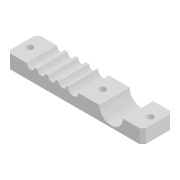
# Autodesk Inventor part: C_Unit_Cable_Holder_B
Saved by Autodesk Inventor 2020 (Build 240168000, 168)
## iProperties
Created: 2021-02-20
Part Number: C_Unit_Cable_Holder_B
Material: 一般
Document SubType Name: Modeling
Designer: ken113
Density: 1 g/cm^3
Appearance: 既定
Author: ken113
Autodesk Inventor part; units mm, degrees
ref_plane "YZ Plane" through (0, 0, 0) normal (1, 0, 0) x (0, 1, 0)
ref_plane "XZ Plane" through (0, 0, 0) normal (0, 1, 0) x (-1, 0, 0)
ref_plane "XY Plane" through (0, 0, 0) normal (0, 0, 1) x (1, 0, 0)
sketch "スケッチ1" plane through (0, 0, 0) normal (0, 0, 1) x (1, 0, 0)
  circle A0 centre (0, 9) radius 7.75
  line L0 (10.75, 0) -> (-58.5, 0)
  line L1 (-58.5, 0) -> (-58.5, 1.25)
  line L2 (-58.5, 1.25) -> (10.75, 1.25)
  line L3 (10.75, 1.25) -> (10.75, 0)
  circle A1 centre (0, 9) radius 10.75
  line L4 (10.75, 1.25) -> (10.75, 15.8822)
  circle A2 centre (-32, 9) radius 2.5
  circle A3 centre (-39, 9) radius 2.5
  circle A4 centre (-25, 9) radius 3.5
  circle A5 centre (-46, 9) radius 2.5
  circle A6 centre (-53, 9) radius 2.5
  circle A7 centre (-53, 9) radius 5.5
  line L5 (-58.5, 1.25) -> (-58.5, 21.0928)
  line L6 (-61.1769, 14.5) -> (16.6826, 14.5)
  point P0 (0, 0)
  point P1 (-9.2365, 14.5)
  point P2 (-58.5, 14.5)
  point P3 (10.75, 14.5)
  point P4 (9.2365, 14.5)
  point P5 (10.75, 9)
  point P6 (5.879, 0)
  point P7 (-5.879, 0)
  dimension "d0" = 15.5
  dimension "d1" = 3
  dimension "d2" = 5
  dimension "d3" = 5
  dimension "d4" = 7
  dimension "d5" = 5
  dimension "d7" = 7
  dimension "d8" = 7
  dimension "d9" = 25
  dimension "d10" = 7
  dimension "d11" = 5
  dimension "d12" = 7
  dimension "d13" = 3
  dimension "d16" = 9
  constraints: 14 end point, 8 centre point, 7 horizontal alignment, 6 tangent, 2 parallel, 2 perpendicular, 1 horizontal, 1 vertical alignment
  measures "d0" diameter of A0
  measures "d1" radial gap between concentric circles of A0 A1
  measures "d2" diameter of A2
  measures "d3" diameter of A3
  measures "d4" diameter of A4
  measures "d5" diameter of A5
  measures "d7" distance of A2.centre A3.centre
  measures "d8" distance of A5.centre A3.centre
  measures "d9" distance of A0.centre A4.centre
  measures "d10" distance of A4.centre A2.centre
  measures "d11" diameter of A6
  measures "d12" distance of A6.centre A5.centre
  measures "d13" radial gap between concentric circles of A6 A7
  measures "d16" distance from line of A4.centre L0
extrude "押し出し1" add sketch "スケッチ1" along normal blind 20 contours A0 L6 A1 L2 | A0 L6 A1 | L2 A1 L6 A0 | L2 A1 L0 | L6 L4 A1 | A1 L0 L1 L2 | L2 L5 A7 A5 L6 A1 | A1 L4 L2 | L2 L3 L0 A1 | A7 A5 | A7 L5 L6 picked at (-49.0972, 10.8197)
sketch "スケッチ3" plane through (0, 0, 20) normal (0, 0, 1) x (1, 0, 0)
  line L0 (-9.2365, 14.5) -> (-58.5, 14.5) projected
  line L1 (-58.5, 14.5) -> (-58.5, 0) projected
  line L2 (-58.5, 0) -> (10.75, 0) projected
  arc A0 (9.2365, 14.5) -> (-9.2365, 14.5) centre (0, 9) ccw projected
  circle A1 centre (0, 9) radius 7.75 projected
  circle A2 centre (-53, 9) radius 2.5 projected
  circle A3 centre (-25, 9) radius 3.5 projected
  circle A4 centre (-39, 9) radius 2.5 projected
  circle A5 centre (-32, 9) radius 2.5 projected
  circle A6 centre (-46, 9) radius 2.5 projected
  line L3 (-58.5, 14.5) -> (-58.5, 0) projected
  line L4 (-58.5, 0) -> (-68.5, 0)
  line L5 (-68.5, 0) -> (-68.5, 14.5)
  line L6 (-68.5, 14.5) -> (-58.5, 14.5)
  line L7 (-58.5, 14.5) -> (-58.5, 0)
  line L8 (10.75, -0.0065) -> (20.75, -0.0065)
  line L9 (20.75, -0.0065) -> (20.75, 14.5)
  line L10 (20.75, 14.5) -> (10.75, 14.5)
  line L11 (10.75, 14.5) -> (10.75, -0.0065)
  line L12 (10.75, 0) -> (10.75, 14.5) projected
  line L13 (10.75, 14.5) -> (9.2365, 14.5) projected
  point P0 (0, 0)
  dimension "d17" = 10
  dimension "d18" = 10
  constraints: 16 end point, 4 parallel, 2 horizontal, 2 perpendicular, 1 coincident, 1 horizontal alignment
  measures "d17" distance of L5.end L6.end
  measures "d18" distance of L10.end L9.end
extrude "押し出し2" add sketch "スケッチ3" against normal up to surface (20 mm away) contours L1 L4 L5 L6 | L10 L9 L8 L11
sketch "スケッチ4" plane through (0, 0, 20) normal (0, 0, 1) x (1, 0, 0)
  line L0 (-9.2365, 14.5) -> (-68.5, 14.5) projected
  line L1 (-68.5, 14.5) -> (-68.5, 0) projected
  line L2 (-68.5, 0) -> (10.75, 0) projected
  line L3 (20.75, -0.0065) -> (20.75, 14.5) projected
  line L4 (20.75, 14.5) -> (9.2365, 14.5) projected
  arc A0 (9.2365, 14.5) -> (-9.2365, 14.5) centre (0, 9) ccw projected
  circle A1 centre (0, 9) radius 7.75 projected
  circle A2 centre (-53, 9) radius 2.5 projected
  circle A3 centre (-25, 9) radius 3.5 projected
  circle A4 centre (-39, 9) radius 2.5 projected
  circle A5 centre (-32, 9) radius 2.5 projected
  circle A6 centre (-46, 9) radius 2.5 projected
  line L5 (-68.5, 0) -> (-68.5, 14.5) projected
  line L6 (-68.5, 9) -> (20.75, 9)
  line L7 (20.75, 9) -> (20.75, 30.4065)
  line L8 (20.75, 30.4065) -> (-68.5, 30.4065)
  line L9 (-68.5, 30.4065) -> (-68.5, 9)
  line L10 (10.75, 0) -> (10.75, -0.0065) projected
  line L11 (10.75, -0.0065) -> (20.75, -0.0065) projected
  point P0 (0, 0)
  point P1 (-55.5, 9)
  point P2 (-40.5, 9)
  point P3 (-48.5, 9)
  point P4 (-33.5, 9)
  point P5 (-41.5, 9)
  point P6 (-26.5, 9)
  point P7 (-34.5, 9)
  point P8 (-19.5, 9)
  point P9 (-18.5, 9)
  point P10 (-21.5, 9)
  point P11 (7.75, 9)
  point P12 (7.75, 9)
  point P13 (10.75, 9)
  point P14 (-21.5, 9)
  point P15 (-28.5, 9)
  point P16 (-29.5, 9)
  point P17 (-29.5, 9)
  point P18 (-36.5, 9)
  point P19 (-36.5, 9)
  point P20 (-43.5, 9)
  point P21 (-43.5, 9)
  point P22 (-50.5, 9)
  point P23 (-50.5, 9)
  point P24 (-68.5, 14.5065)
  point P25 (20.75, 14.5)
  point P26 (-68.5, 14.5)
  point P27 (20.75, 14.5)
  constraints: 6 end point, 1 horizontal, 1 horizontal alignment, 1 parallel, 1 point on line, 1 vertical, 3 other
extrude "押し出し3" cut sketch "スケッチ4" against normal through all contours A0 L4 L3 L6 A1 A3 A5 A4 A6 A2 L1 L0 | L0 L9 L8 L7 L4 A0 | A2 L6 | L6 A1 | A6 L6 | L6 A3 | A4 L6 | L6 A5 picked at (-52.3762, 9.5526) picked at (1.4675, 11.126) picked at (-45.3762, 9.5526) picked at (-24.5863, 10.0909) picked at (-38.3762, 9.5526) picked at (-32.7192, 9.9399)
sketch "スケッチ6" plane through (7.75, 9, 20) normal (0, 1, 0) x (1, 0, 0)
  line L0 (0, 0) -> (0, 20) projected
  line L1 (13, 0) -> (0, 0) projected
  line L2 (13, 20) -> (13, 0) projected
  line L3 (-29.25, 0) -> (-29.25, 20) projected
  line L4 (-15.5, 0) -> (-29.25, 0) projected
  line L5 (-15.5, 20) -> (-15.5, 0) projected
  line L6 (-63.25, 20) -> (-63.25, 0) projected
  line L7 (-76.25, 0) -> (-76.25, 20) projected
  line L8 (-63.25, 0) -> (-76.25, 0) projected
  line L9 (-76.25, 20) -> (-63.25, 20) projected
  line L10 (-29.25, 20) -> (-15.5, 20) projected
  line L11 (0, 20) -> (13, 20) projected
  point P0 (-7.75, 20)
  point P1 (8, 10)
  point P2 (-23.5, 10)
  point P3 (-71.25, 10)
  dimension "d33" = 10
  dimension "d34" = 5
  dimension "d35" = 5
  dimension "d36" = 15.75
  constraints: 2 horizontal alignment
  measures "d33" distance from line of L1 point (8, 10)
  measures "d34" distance from line of point (8, 10) L2
  measures "d35" distance from line of L7 point (-71.25, 10)
  measures "d36" horizontal distance of point (-23.5, 10) point (-7.75, 20)
hole "穴2" at (15.75, 9, 10) at (-15.75, 9, 10) at (-63.5, 9, 10) direction (0, -1, 0) diameter 4.3 end through all
chamfer "面取り1" distance 2 angle 45 4 edges at (20.75, 4.4968, 0) (20.75, 4.4968, 20) (-68.5, 4.5, 0) (-68.5, 4.5, 20)
